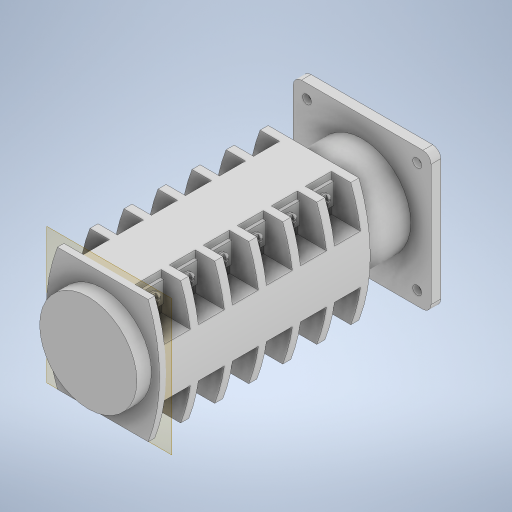
# Autodesk Inventor part: Parte6
Saved by Autodesk Inventor 2024 (Build 280153000, 153)
## iProperties
Created: 2023-12-18
Part Number: Parte6
Material: Generico
Document SubType Name: Modeling
Designer: cecca
Density: 1 g/cm^3
Appearance: Default
Author: cecca
Autodesk Inventor part; units mm, degrees
ref_plane "YZ Plane" through (0, 0, 0) normal (1, 0, 0) x (0, 1, 0)
ref_plane "XZ Plane" through (0, 0, 0) normal (0, 1, 0) x (-1, 0, 0)
ref_plane "XY Plane" through (0, 0, 0) normal (0, 0, 1) x (1, 0, 0)
sketch "Schizzo1" plane through (0, 0, 0) normal (0, 0, 1) x (1, 0, 0)
  circle A0 centre (0, 0) radius 30
  dimension "d0" = 60
  constraints: 1 centre point, 1 coincident
  measures "d0" diameter of A0
extrude "Estrusione1" add sketch "Schizzo1" along normal mid plane 30
sketch "Schizzo2" plane through (0, 0, 15) normal (0, 0, 1) x (1, 0, 0)
  line L0 (38, -35) -> (-38, 35) construction
  line L1 (-38, -35) -> (38, 35) construction
  line L2 (35, 38) -> (-35, 38)
  line L3 (-35, 38) -> (-35, -38)
  line L4 (-35, -38) -> (35, -38)
  line L5 (35, -38) -> (35, 38)
  line L6 (35, 38) -> (-35, -38) construction
  line L7 (-35, 38) -> (35, -38) construction
  point P0 (0, 0)
  dimension "d11" = 70
  dimension "d12" = 76
  constraints: 16 end point, 4 midpoint, 2 parallel, 1 horizontal, 1 perpendicular
  measures "d11" distance of L4.end L3.end
  measures "d12" distance of L3.end L2.end
extrude "Estrusione2" add sketch "Schizzo2" along normal blind 130
sketch "Schizzo5" plane through (0, 0, 145) normal (0, 0, 1) x (1, 0, 0)
  circle A0 centre (0, 0) radius 30
  dimension "d13" = 60
  constraints: 1 centre point, 1 coincident
  measures "d13" diameter of A0
extrude "Estrusione4" add sketch "Schizzo5" along normal blind 9
sketch "Schizzo6" plane through (0, 0, 145) normal (0, 0, 1) x (1, 0, 0)
  line L0 (35, 38) -> (-35, 38) projected
  line L1 (-35, 38) -> (-28, 38)
  line L2 (35, -38) -> (35, 38) projected
  line L3 (35, 38) -> (28, 38)
  line L4 (-28, -38) -> (28, -38)
  line L5 (28, -38) -> (28, 38)
  line L6 (28, 38) -> (-28, 38)
  line L7 (-28, 38) -> (-28, -38)
  line L8 (-28, -38) -> (28, 38) construction
  line L9 (28, -38) -> (-28, 38) construction
  line L10 (35, 0) -> (71.643, 0)
  circle A0 centre (71.643, 0) radius 106.643
  line L11 (0, -150.7603) -> (0, 206.7907)
  circle A1 centre (-71.643, 0) radius 106.643
  point P0 (0, 0)
  point P1 (0, -78.9937)
  point P2 (0, 78.9937)
  dimension "d17" = 7
  dimension "d18" = 7
  dimension "d19" = 36.643
  constraints: 20 end point, 3 midpoint, 2 horizontal, 2 parallel, 2 point on line, 1 centre point, 1 coincident, 1 perpendicular, 1 symmetric about line, 1 vertical, 4 other
  measures "d17" distance of L0.end L1.end
  measures "d18" distance of L0.start L3.end
  measures "d19" distance of L10.start L10.end
extrude "Estrusione5" cut sketch "Schizzo6" along normal mid plane 320 contours L2 A1 L0 | L0 A1 A0 L2 | A0 A1
ref_plane "Piano di lavoro1" through (0, 0, 141) normal (0, 0, 1) x (1, 0, 0)
sketch "Schizzo7" plane through (0, 0, 141) normal (0, 0, 1) x (1, 0, 0)
  line L0 (0, 0) -> (-16, 0)
  line L1 (-32, 15) -> (-32, -15)
  line L2 (-32, -15) -> (-16, -15)
  line L3 (-16, 15) -> (-16, 51.246)
  line L4 (-16, 51.246) -> (-49.061, 51.246)
  line L5 (-16, -15) -> (-16, -51.246)
  line L6 (-16, -51.246) -> (-49.061, -51.246)
  line L7 (-49.061, -51.246) -> (-49.061, 51.246)
  line L8 (-16, -15) -> (-38, -15)
  line L9 (-38, -15) -> (-38, 15)
  line L10 (-38, 15) -> (-16, 15)
  dimension "d25" = 30
  dimension "d27" = 36.246
  dimension "d28" = 33.061
  dimension "d29" = 36.246
  dimension "d30" = 33.061
  dimension "d31" = 22
  constraints: 22 end point, 3 perpendicular, 2 horizontal, 1 parallel, 1 point on line, 1 vertical
  measures "d25" distance of L2.end L3.start
  measures "d27" distance of L3.start L3.end
  measures "d28" distance of L3.end L4.end
  measures "d29" distance of L2.end L5.end
  measures "d30" distance of L5.end L6.end
  measures "d31" distance of L2.end L8.end
extrude "Estrusione6" cut sketch "Schizzo7" against normal blind 16 contours L10 L9 L8 L2 L5 L6 L7 L4 L3
pattern_linear "Serie rettangolare1" count 6 spacing 21 along (0, 0, -1) of "Estrusione6"
mirror "Speculare1" about plane through (0, 0, 0) normal (1, 0, 0) of "Estrusione6", "Serie rettangolare1"
sketch "Schizzo8" plane through (0, 0, -15) normal (0, 0, -1) x (-1, 0, 0)
  line L0 (-42.5, -42.5) -> (42.5, -42.5)
  line L1 (42.5, -42.5) -> (42.5, 42.5)
  line L2 (42.5, 42.5) -> (-42.5, 42.5)
  line L3 (-42.5, 42.5) -> (-42.5, -42.5)
  line L4 (-42.5, -42.5) -> (42.5, 42.5) construction
  line L5 (42.5, -42.5) -> (-42.5, 42.5) construction
  point P0 (0, 0)
  dimension "d37" = 85
  dimension "d38" = 85
  constraints: 12 end point, 2 midpoint, 2 parallel, 1 horizontal, 1 perpendicular
  measures "d37" distance of L2.end L1.end
  measures "d38" distance of L1.end L0.end
extrude "Estrusione7" add sketch "Schizzo8" along normal blind 6
fillet "Raccordo1" radius 5 4 edges at (-42.5, -42.5, -18) (-42.5, 42.5, -18) (42.5, -42.5, -18) (42.5, 42.5, -18)
sketch "Schizzo9" plane through (-16, -38, 141) normal (-1, 0, 0) x (0, 0, 1)
  line L0 (0, 0) -> (0, 23) projected
  line L1 (-16, 0) -> (-21, 0) projected
  line L2 (0, 23) -> (-16, 23)
  line L3 (-16, 23) -> (-16, 0)
  line L4 (-16, 0) -> (0, 0)
  line L5 (0, 0) -> (0, 23)
  line L6 (-8, 4) -> (-15.5, 4)
  line L7 (-15.5, 4) -> (-15.5, 17)
  line L8 (-15.5, 17) -> (-0.5, 17)
  line L9 (-0.5, 17) -> (-0.5, 4)
  line L10 (-0.5, 4) -> (-8, 4)
  point P0 (-141, 38)
  dimension "d45" = 7.5
  dimension "d46" = 13
  dimension "d47" = 15
  constraints: 18 end point, 5 perpendicular, 3 parallel, 1 horizontal, 1 point on line
  measures "d45" distance of L6.start L6.end
  measures "d46" distance of L6.end L7.end
  measures "d47" distance of L7.end L8.end
extrude "Estrusione8" add sketch "Schizzo9" along normal blind 2 contours L6 L7 L8 L9 L10
sketch "Schizzo10" plane through (-18, -38, 141) normal (-1, 0, 0) x (0, 0, 1)
  line L0 (-15.5, 17) -> (-15.5, 4) projected
  line L1 (-15.5, 4) -> (-8, 4)
  line L2 (-15.5, 4) -> (-0.5, 4) projected
  circle A0 centre (-8, 10.5) radius 4
  point P0 (-141, 38)
  dimension "d50" = 7.5
  dimension "d52" = 8
  constraints: 2 end point, 1 centre point, 1 midpoint
  measures "d50" distance of L0.end L1.end
  measures "d52" diameter of A0
extrude "Estrusione9" add sketch "Schizzo10" along normal blind 3
fillet "Raccordo2" radius 2 1 edges at (-21, -27.5, 129)
sketch "Schizzo11" plane through (-21, -27.5, 133) normal (-1, 0, 0) x (0, 0, 1)
  circle A0 centre (0, 0) radius 4
  line L0 (0.75, 5) -> (-0.75, 5)
  line L1 (-0.75, 5) -> (-0.75, -5)
  line L2 (-0.75, -5) -> (0.75, -5)
  line L3 (0.75, -5) -> (0.75, 5)
  line L4 (0.75, 5) -> (-0.75, -5) construction
  line L5 (-0.75, 5) -> (0.75, -5) construction
  line L6 (-5, -0.75) -> (5, -0.75)
  line L7 (5, -0.75) -> (5, 0.75)
  line L8 (5, 0.75) -> (-5, 0.75)
  line L9 (-5, 0.75) -> (-5, -0.75)
  line L10 (-5, -0.75) -> (5, 0.75) construction
  line L11 (5, -0.75) -> (-5, 0.75) construction
  point P0 (-133, 27.5)
  point P1 (-0.75, -0.75)
  point P2 (-0.75, -3.9291)
  point P3 (0.75, -3.9291)
  point P4 (0.75, -0.75)
  point P5 (3.9291, -0.75)
  point P6 (3.9291, 0.75)
  point P7 (0.75, 0.75)
  point P8 (0.75, 3.9291)
  point P9 (-0.75, 3.9291)
  point P10 (-0.75, 0.75)
  point P11 (-3.9291, 0.75)
  point P12 (-3.9291, -0.75)
  dimension "d56" = 1.5
  dimension "d57" = 10
  dimension "d58" = 10
  dimension "d59" = 1.5
  constraints: 24 end point, 4 midpoint, 4 parallel, 2 horizontal, 2 perpendicular, 1 centre point
  measures "d56" distance of L2.end L1.end
  measures "d57" distance of L1.end L0.end
  measures "d58" distance of L8.end L7.end
  measures "d59" distance of L7.end L6.end
extrude "Estrusione10" cut sketch "Schizzo11" against normal blind 1 contours A0 L6 L3 L8 | L3 L8 L1 A0 | L3 L6 L1 L8 | A0 L1 L6 L3 | L1 L6 A0 L8
pattern_linear "Serie rettangolare2" count 6 spacing 21 along (0, 0, -1) of "Estrusione10", "Raccordo2", "Estrusione9", "Estrusione8"
mirror "Speculare2" about plane through (0, 0, 0) normal (0, 1, 0) of "Estrusione8", "Estrusione9", "Estrusione10", "Raccordo2", "Serie rettangolare2"
mirror "Speculare3" about plane through (0, 0, 0) normal (1, 0, 0) of "Estrusione8", "Estrusione9", "Estrusione10", "Raccordo2", "Serie rettangolare2", "Speculare2"
sketch "Schizzo12" plane through (0, 0, -21) normal (0, 0, -1) x (-1, 0, 0)
  circle A0 centre (0, 0) radius 12
  dimension "d65" = 24
  constraints: 1 centre point, 1 coincident
  measures "d65" diameter of A0
extrude "Estrusione11" cut sketch "Schizzo12" against normal blind 5
sketch "Schizzo13" plane through (0, 0, -16) normal (0, 0, -1) x (-1, 0, 0)
  line L0 (0, 0) -> (7.506, 0)
  line L1 (0, 0) -> (-7.506, 0)
  line L2 (0, 0) -> (0, 6.5)
  line L3 (0, 0) -> (0, -6.5)
  line L4 (0, 6.5) -> (-3.753, 6.5)
  line L5 (0, 6.5) -> (3.753, 6.5)
  line L6 (3.753, 6.5) -> (7.506, 0)
  line L7 (-3.753, 6.5) -> (-7.506, 0)
  line L8 (0, -6.5) -> (-3.753, -6.5)
  line L9 (0, -6.5) -> (3.753, -6.5)
  line L10 (3.753, -6.5) -> (7.506, 0)
  line L11 (-3.753, -6.5) -> (-7.506, 0)
  dimension "d68" = 7.506
  dimension "d69" = 7.506
  dimension "d70" = 6.5
  dimension "d71" = 6.5
  dimension "d72" = 3.753
  dimension "d73" = 3.753
  constraints: 24 end point, 4 horizontal, 2 symmetric about line, 2 vertical
  measures "d68" distance of L0.start L0.end
  measures "d69" distance of L0.start L1.end
  measures "d70" distance of L0.start L2.end
  measures "d71" distance of L0.start L3.end
  measures "d72" distance of L2.end L4.end
  measures "d73" distance of L2.end L5.end
extrude "Estrusione12" add sketch "Schizzo13" along normal blind 37
sketch "Schizzo14" plane through (0, 0, -53) normal (0, 0, -1) x (-1, 0, 0)
  line L0 (7.506, 0) -> (3.753, 6.5) projected
  line L1 (7.506, 0) -> (-5.494, 0)
  line L2 (-5.494, 0) -> (-5.494, 18.7866)
  line L3 (-5.494, 18.7866) -> (7.506, 18.7866)
  line L4 (7.506, 18.7866) -> (7.506, 0)
  line L5 (7.506, 0) -> (-5.494, 0)
  line L6 (-5.494, 0) -> (-5.494, -13.8572)
  line L7 (-5.494, -13.8572) -> (7.506, -13.8572)
  line L8 (7.506, -13.8572) -> (7.506, 0)
  line L9 (-5.494, -5.7954) -> (-8.5353, -5.7954)
  line L10 (-8.5353, -5.7954) -> (-8.5353, 4.9557)
  line L11 (-8.5353, 4.9557) -> (-5.494, 4.9557)
  line L12 (-5.494, 4.9557) -> (-5.494, -5.7954)
  point P0 (0, 0)
  dimension "d76" = 13
  constraints: 24 end point, 6 parallel, 3 horizontal, 3 perpendicular, 2 point on line
  measures "d76" distance of L2.end L3.end
extrude "Estrusione13" cut sketch "Schizzo14" against normal blind 15 contours L6 L9 L10 L11 L2
sketch "Schizzo15" plane through (0, 0, -21) normal (0, 0, -1) x (-1, 0, 0)
  line L0 (34, -34) -> (-34, -34)
  line L1 (-34, -34) -> (-34, 34)
  line L2 (-34, 34) -> (34, 34)
  line L3 (34, 34) -> (34, -34)
  line L4 (34, -34) -> (-34, 34) construction
  line L5 (-34, -34) -> (34, 34) construction
  point P0 (0, 0)
  dimension "d79" = 68
  dimension "d80" = 68
  constraints: 12 end point, 2 midpoint, 2 parallel, 1 horizontal, 1 perpendicular
  measures "d79" distance of L1.end L2.end
  measures "d80" distance of L0.end L1.end
hole "Foro1" at (34, 34, -21) at (-34, 34, -21) at (-34, -34, -21) at (34, -34, -21) direction (0, 0, 1) diameter 5.5 end through all countersink diameter 10.4 countersink angle 90 clearance for "Vite a testa svasata piana ISO 2009/7046" size "M5" standard "ISO"
